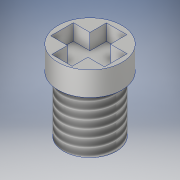
# Autodesk Inventor part: sqrew for baring stand
Saved by Autodesk Inventor 2018 (Build 220112000, 112)
## iProperties
Created: 2018-03-02
Part Number: sqrew for baring stand
Material: Aluminum 6061
Document SubType Name: Modeling
Designer: 238438
Density: 2.7 g/cm^3
Appearance: Aluminum - Flat
Mass: 0.229255 g
Surface Area: 1.51361 cm^2
Volume: 0.0849094 cm^3
Author: 238438
Autodesk Inventor part; units mm, degrees
ref_plane "YZ Plane" through (0, 0, 0) normal (1, 0, 0) x (0, 1, 0)
ref_plane "XZ Plane" through (0, 0, 0) normal (0, 1, 0) x (-1, 0, 0)
ref_plane "XY Plane" through (0, 0, 0) normal (0, 0, 1) x (1, 0, 0)
sketch "Sketch1" plane through (0, 0, 0) normal (0, 0, 1) x (1, 0, 0)
  line L0 (0, 0) -> (2.54, 0)
  line L1 (2.54, 0) -> (2.54, -1.905)
  line L2 (2.54, -1.905) -> (2.0955, -1.905)
  line L3 (2.0955, -1.905) -> (2.0955, -6.35)
  line L4 (2.0955, -6.35) -> (0, -6.35)
  line L5 (0, -6.35) -> (0, 0)
  line L6 (0, 0) -> (0, -8.8327)
  dimension "d0" = 2.54
  dimension "d1" = 1.905
  dimension "d2" = 0.4445
  dimension "d3" = 4.445
  constraints: 14 end point, 3 perpendicular, 2 horizontal, 1 point on line, 1 vertical
  measures "d0" distance of L0.start L0.end
  measures "d1" distance of L0.end L1.end
  measures "d2" distance of L1.end L2.end
  measures "d3" distance of L2.end L3.end
revolve "Revolution1" add sketch "Sketch1" angle 360 about axis through (0, 0, 0) along (0, -1, 0)
thread "Thread1" size "5-40 UNC" class "2A" standard "ANSI Unified Screw Threads" full length
sketch "Sketch2" plane through (0, 0, 0) normal (0, 1, 0) x (1, 0, 0)
  line L0 (2.1608, 0.7916) -> (2.1608, -1.0055)
  line L1 (-2.1181, -1.0055) -> (-2.1181, 0.7916)
  line L2 (-0.7916, 2.0955) -> (0.8344, 2.0955)
  line L3 (0.8344, -2.2464) -> (-0.7916, -2.2464)
  line L4 (-0.7916, -2.2464) -> (-0.7916, -1.0055)
  line L5 (-0.7916, 0.7916) -> (-0.7916, 2.0955)
  line L6 (-2.1181, 0.7916) -> (-0.7916, 0.7916)
  line L7 (0.8344, 0.7916) -> (2.1608, 0.7916)
  line L8 (0.8344, 2.0955) -> (0.8344, 0.7916)
  line L9 (0.8344, -1.0055) -> (0.8344, -2.2464)
  line L10 (2.1608, -1.0055) -> (0.8344, -1.0055)
  line L11 (-0.7916, -1.0055) -> (-2.1181, -1.0055)
  point P0 (0, 0)
  constraints: 24 end point, 10 parallel, 4 perpendicular, 3 horizontal
extrude "Extrusion1" cut sketch "Sketch2" against normal blind 1.27
body "Solid1"
